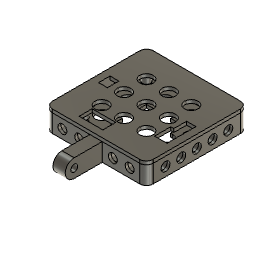
USB Camera Case v10 (Autodesk Fusion 360 design; units mm, degrees)
Autodesk Fusion 360 part; units mm, degrees
note: some values were not read from the file. Chosen so that the rebuilt part matches the saved one: which bodies a step acts on; which face or edge a step refers to. Set by a fixed rule: which sketch regions a step uses.
sketch "Camer Cutout" plane through (0, 0, 0) normal (0, 0, 1) x (1, 0, 0)
  line L0 (8.25, -8.25) -> (-8.25, -8.25)
  line L1 (-8.25, -8.25) -> (-8.25, 8.25)
  line L2 (-8.25, 8.25) -> (8.25, 8.25)
  line L3 (8.25, 8.25) -> (8.25, -8.25)
  line L4 (8.25, -8.25) -> (-8.25, 8.25) construction
  line L5 (-8.25, -8.25) -> (8.25, 8.25) construction
  arc A0 (8.25, -2.5) -> (8.25, 2.5) centre (8.25, 0) ccw
  arc A1 (-8.25, 2.5) -> (-8.25, -2.5) centre (-8.25, 0) ccw
  dimension "d1" = 16.5
  dimension "d2" = 16.5
  dimension "d3" = 2.5
  dimension "d4" = 2.5
  constraint horizontal L0
  constraint perpendicular L0 L1
  constraint parallel L0 L2
  constraint parallel L1 L3
  constraint coincident L4 origin
  constraint coincident L5 origin
  constraint midpoint L3 A0.centre
  constraint midpoint L1 A1.centre
  measures "d1" distance of L1.end L2.end
  measures "d2" distance of L0.end L1.end
  measures "d3" radius of A0
  measures "d4" radius of A1
sketch "Outer Standoff Lines" plane through (0, 0, 0) normal (0, 0, 1) x (1, 0, 0)
  line L0 (0, 0) -> (17, 0)
  line L1 (0, 0) -> (-17, 0)
  line L2 (-17, 0) -> (-17, 17)
  line L3 (-17, 0) -> (-17, -17)
  line L4 (17, 0) -> (17, -17)
  line L5 (17, 0) -> (17, 17)
  dimension "d5" = 17
  dimension "d6" = 17
  dimension "d7" = 17
  dimension "d8" = 17
  dimension "d9" = 17
  constraint coincident L0.start L1.start
  constraint horizontal L0
  constraint parallel L0 L1
  constraint perpendicular L1 L2
  constraint perpendicular L1 L3
  constraint perpendicular L0 L4
  constraint perpendicular L0 L5
  measures "d5" distance of L0.start L0.end
  measures "d6" distance of L1.end L2.end
  measures "d7" distance of L1.end L3.end
  measures "d8" distance of L0.end L4.end
  measures "d9" distance of L0.end L5.end
sketch "Inner Standoff Lines" plane through (0, 0, 0) normal (0, 0, 1) x (1, 0, 0)
  line L0 (0, 0) -> (14, 0)
  line L1 (14, 0) -> (14, -14)
  line L2 (14, 0) -> (14, 14)
  line L3 (0, 0) -> (-14, 0)
  line L4 (-14, 0) -> (-14, 14)
  line L5 (-14, 0) -> (-14, -14)
  dimension "d10" = 14
  dimension "d11" = 14
  dimension "d12" = 14
  dimension "d13" = 14
  dimension "d14" = 14
  dimension "d15" = 14
  constraint coincident L0.start L3.start
  constraint horizontal L0
  constraint perpendicular L0 L1
  constraint perpendicular L0 L2
  constraint perpendicular L2 L3
  constraint perpendicular L3 L4
  constraint perpendicular L3 L5
  measures "d10" distance of L0.start L0.end
  measures "d11" distance of L0.end L1.end
  measures "d12" distance of L0.end L2.end
  measures "d13" distance of L0.start L3.end
  measures "d14" distance of L3.end L4.end
  measures "d15" distance of L3.end L5.end
sketch "Outer Standoffs" plane through (0, 0, 0) normal (0, 0, 1) x (1, 0, 0)
  circle A0 centre (-17, 17) radius 1.1
  circle A1 centre (-17, -17) radius 1.1
  circle A2 centre (17, -17) radius 1.1
  circle A3 centre (17, 17) radius 1.1
  dimension "d16" = 2.2
  dimension "d17" = 2.2
  dimension "d18" = 2.2
  dimension "d19" = 2.2
  measures "d16" diameter of A0
  measures "d17" diameter of A1
  measures "d18" diameter of A2
  measures "d19" diameter of A3
sketch "Inner Standoffs" plane through (0, 0, 0) normal (0, 0, 1) x (1, 0, 0)
  circle A0 centre (-14, 14) radius 1.1
  circle A1 centre (-14, -14) radius 1.1
  circle A2 centre (14, -14) radius 1.1
  circle A3 centre (14, 14) radius 1.1
  dimension "d20" = 2.2
  dimension "d21" = 2.2
  dimension "d22" = 2.2
  dimension "d23" = 2.2
  measures "d20" diameter of A0
  measures "d21" diameter of A1
  measures "d22" diameter of A2
  measures "d23" diameter of A3
sketch "Inner Standoff Bases" plane through (0, 0, 0) normal (0, 0, 1) x (1, 0, 0)
  circle A0 centre (-14, 14) radius 1.75
  circle A1 centre (-14, -14) radius 1.75
  circle A2 centre (14, -14) radius 1.75
  circle A3 centre (14, 14) radius 1.75
  dimension "d24" = 3.5
  dimension "d25" = 3.5
  dimension "d26" = 3.5
  dimension "d27" = 3.5
  measures "d24" diameter of A0
  measures "d25" diameter of A1
  measures "d26" diameter of A2
  measures "d27" diameter of A3
sketch "Outer Standoff Bases" plane through (0, 0, 0) normal (0, 0, 1) x (1, 0, 0)
  circle A0 centre (-17, 17) radius 1.75
  circle A1 centre (-17, -17) radius 1.75
  circle A2 centre (17, -17) radius 1.75
  circle A3 centre (17, 17) radius 1.75
  dimension "d28" = 3.5
  dimension "d29" = 3.5
  dimension "d30" = 3.5
  dimension "d31" = 3.5
  measures "d28" diameter of A0
  measures "d29" diameter of A1
  measures "d30" diameter of A2
  measures "d31" diameter of A3
sketch "Board Cutout" plane through (0, 0, 0) normal (0, 0, 1) x (1, 0, 0)
  line L0 (19.15, 19.15) -> (-19.15, 19.15)
  line L1 (-19.15, 19.15) -> (-19.15, -19.15)
  line L2 (-19.15, -19.15) -> (19.15, -19.15)
  line L3 (19.15, -19.15) -> (19.15, 19.15)
  line L4 (19.15, 19.15) -> (-19.15, -19.15) construction
  line L5 (-19.15, 19.15) -> (19.15, -19.15) construction
  dimension "d32" = 38.3
  dimension "d33" = 38.3
  constraint horizontal L0
  constraint perpendicular L0 L1
  constraint parallel L0 L2
  constraint parallel L1 L3
  constraint coincident L4 origin
  constraint coincident L5 origin
  measures "d32" distance of L1.end L2.end
  measures "d33" distance of L0.end L1.end
sketch "Case Outer Footprint" plane through (0, 0, 0) normal (0, 0, 1) x (1, 0, 0)
  line L0 (19.5, -22.5) -> (-19.5, -22.5)
  line L1 (-22.5, -19.5) -> (-22.5, 19.5)
  line L2 (-19.5, 22.5) -> (19.5, 22.5)
  line L3 (22.5, 19.5) -> (22.5, -19.5)
  line L4 (22.5, -22.5) -> (-22.5, 22.5) construction
  line L5 (-22.5, -22.5) -> (22.5, 22.5) construction
  arc A0 (-19.5, 22.5) -> (-22.5, 19.5) centre (-19.5, 19.5) ccw
  arc A1 (-22.5, -19.5) -> (-19.5, -22.5) centre (-19.5, -19.5) ccw
  arc A2 (19.5, -22.5) -> (22.5, -19.5) centre (19.5, -19.5) ccw
  arc A3 (22.5, 19.5) -> (19.5, 22.5) centre (19.5, 19.5) ccw
  dimension "d34" = 45
  dimension "d35" = 45
  dimension "d36" = 3
  constraint horizontal L0
  constraint perpendicular L0 L1
  constraint parallel L0 L2
  constraint parallel L1 L3
  constraint coincident L4 origin
  constraint coincident L5 origin
  constraint coincident L4.end L2
  constraint coincident L4.end L1
  constraint tangent L2 A0
  constraint tangent L1 A0
  constraint coincident L5.start L1
  constraint coincident L5.start L0
  constraint tangent L1 A1
  constraint tangent L0 A1
  constraint equal A0 A1
  constraint coincident L4.start L0
  constraint coincident L4.start L3
  constraint tangent L0 A2
  constraint tangent L3 A2
  constraint equal A0 A2
  constraint coincident L5.end L3
  constraint coincident L5.end L2
  constraint tangent L3 A3
  constraint tangent L2 A3
  constraint equal A0 A3
  measures "d34" distance of L4.end L5.end
  measures "d35" distance of L5.start L4.end
  measures "d36" radius of A0
sketch "Port 2 Cutout" plane through (0, 0, 0) normal (0, 0, 1) x (1, 0, 0)
  line L0 (-14, -14) -> (-10.5, -14)
  line L1 (-10.5, -14) -> (-10.5, -19.15)
  line L2 (-10.5, -19.15) -> (-10.5, -14.25)
  line L3 (-10.5, -14.25) -> (-0.35, -14.25)
  line L4 (-0.35, -14.25) -> (-0.35, -19.15)
  line L5 (-0.35, -19.15) -> (-10.5, -19.15)
  dimension "d37" = 3.5
  dimension "d38" = 5.15
  dimension "d39" = 4.9
  dimension "d40" = 10.15
  dimension "d41" = 4.9
  constraint horizontal L0
  constraint vertical L1
  constraint perpendicular L0 L2
  constraint perpendicular L2 L3
  constraint perpendicular L3 L4
  measures "d37" distance of L0.start L0.end
  measures "d38" distance of L0.end L1.end
  measures "d39" distance of L1.end L2.end
  measures "d40" distance of L2.end L3.end
  measures "d41" distance of L3.end L4.end
sketch "Port 1 Cutout" plane through (0, 0, 0) normal (0, 0, 1) x (1, 0, 0)
  line L0 (-14, -14) -> (-14, -1.8)
  line L1 (-14, -1.8) -> (-19.15, -1.8)
  line L2 (-19.15, -1.8) -> (-19.15, 2.9)
  line L3 (-19.15, 2.9) -> (-15.65, 2.9)
  line L4 (-15.65, 2.9) -> (-15.65, -1.8)
  dimension "d42" = 12.2
  dimension "d43" = 5.15
  dimension "d44" = 4.7
  dimension "d45" = 3.5
  constraint vertical L0
  constraint perpendicular L0 L1
  constraint perpendicular L1 L2
  constraint perpendicular L2 L3
  constraint coincident L1 L4.end
  constraint perpendicular L1 L4
  measures "d42" distance of L0.start L0.end
  measures "d43" distance of L0.end L1.end
  measures "d44" distance of L1.end L2.end
  measures "d45" distance of L2.end L3.end
sketch "Ports 3/4 Cutout" plane through (0, 0, 0) normal (0, 0, 1) x (1, 0, 0)
  line L0 (14, -14) -> (14, -10)
  line L1 (14, -10) -> (19.15, -10)
  line L2 (14, -10) -> (14, -3)
  line L3 (19.15, -10) -> (19.15, 2.5)
  line L4 (14, -3) -> (15.4, -3)
  line L5 (15.4, -3) -> (15.4, 2.5)
  line L6 (15.4, 2.5) -> (19.15, 2.5)
  dimension "d46" = 4
  dimension "d47" = 5.15
  dimension "d48" = 7
  dimension "d49" = 12.5
  dimension "d50" = 1.4
  constraint vertical L0
  constraint perpendicular L0 L1
  constraint perpendicular L1 L2
  constraint perpendicular L1 L3
  constraint perpendicular L2 L4
  constraint perpendicular L4 L5
  constraint perpendicular L3 L6
  measures "d46" distance of L0.start L0.end
  measures "d47" distance of L0.end L1.end
  measures "d48" distance of L0.end L2.end
  measures "d49" distance of L1.end L3.end
  measures "d50" distance of L2.end L4.end
sketch "Back Insert Footprint" plane through (0, 0, 0) normal (0, 0, 1) x (1, 0, 0)
  line L0 (18.75, 21.25) -> (-18.75, 21.25)
  line L1 (-21.25, 18.75) -> (-21.25, -18.75)
  line L2 (-18.75, -21.25) -> (18.75, -21.25)
  line L3 (21.25, -18.75) -> (21.25, 18.75)
  line L4 (21.25, 21.25) -> (-21.25, -21.25) construction
  line L5 (-21.25, 21.25) -> (21.25, -21.25) construction
  arc A0 (-18.75, 21.25) -> (-21.25, 18.75) centre (-18.75, 18.75) ccw
  arc A1 (-21.25, -18.75) -> (-18.75, -21.25) centre (-18.75, -18.75) ccw
  arc A2 (18.75, -21.25) -> (21.25, -18.75) centre (18.75, -18.75) ccw
  arc A3 (21.25, 18.75) -> (18.75, 21.25) centre (18.75, 18.75) ccw
  dimension "d51" = 42.5
  dimension "d52" = 42.5
  dimension "d53" = 2.5
  constraint horizontal L0
  constraint perpendicular L0 L1
  constraint parallel L0 L2
  constraint parallel L1 L3
  constraint coincident L4 origin
  constraint coincident L5 origin
  constraint coincident L5.start L0
  constraint coincident L5.start L1
  constraint tangent L0 A0
  constraint tangent L1 A0
  constraint coincident L4.end L1
  constraint coincident L4.end L2
  constraint tangent L1 A1
  constraint tangent L2 A1
  constraint equal A0 A1
  constraint coincident L5.end L2
  constraint coincident L5.end L3
  constraint tangent L2 A2
  constraint tangent L3 A2
  constraint equal A0 A2
  constraint coincident L4.start L3
  constraint coincident L4.start L0
  constraint tangent L3 A3
  constraint tangent L0 A3
  constraint equal A0 A3
  measures "d51" distance of L4.end L5.end
  measures "d52" distance of L5.start L4.end
  measures "d53" radius of A0
extrude "Extrude1" add sketch "Case Outer Footprint" along normal blind 8 makes body 1
extrude "Extrude2" cut sketch "Back Insert Footprint" along normal blind 20 from surface at 1.5 bodies 1
extrude "Extrude3" cut sketch "Camer Cutout" along normal blind 5 bodies 1
extrude "Extrude4" add sketch "Outer Standoff Bases" sketch "Inner Standoff Bases" along normal blind 3 of sketch 2 bodies 1
extrude "Extrude5" add sketch "Inner Standoffs" sketch "Outer Standoffs" along normal blind 5.5 of sketch 2 bodies 1
extrude "Extrude6" add sketch "Outer Standoff Bases" sketch "Inner Standoff Bases" along normal blind 3.3 from surface at 4.7 separate body of sketch 2 makes body 2 at (-12.2587, 13.8258, 5.8) makes body 3 at (15.7413, 13.8258, 5.8) makes body 4 at (-15.2587, 16.8258, 5.8) makes body 5 at (18.7413, 16.8258, 5.8) makes body 6 at (-15.2587, -17.1742, 5.8) makes body 7 at (18.7413, -17.1742, 5.8) makes body 8 at (-12.2587, -14.1742, 5.8) makes body 9 at (15.7413, -14.1742, 5.8)
extrude "Extrude7" add sketch "Case Outer Footprint" along normal blind 1.5 from surface at 8 bodies 2 3 4 5 6 7 8 9
extrude "Extrude8" cut sketch "Inner Standoffs" sketch "Outer Standoffs" along normal blind 5.5 of sketch 2 bodies 2
extrude "Extrude9" cut sketch "Ports 3/4 Cutout" sketch "Port 1 Cutout" sketch "Port 2 Cutout" along normal blind 10 of sketch 2 of sketch 3 bodies 2
extrude "Extrude10" add sketch "Back Insert Footprint" sketch "Board Cutout" along normal blind 8 separate body of sketch 2 makes body 10
extrude "Extrude11" cut sketch "Board Cutout" along normal blind 8 bodies 10
extrude "Extrude12" cut sketch "Back Insert Footprint" along normal blind 1.5 bodies 10
combine "Combine1" operation add target body 2 tool bodies 10
sketch "Mount Arm" plane through (0, 0, 0) normal (1, 0, 0) x (0, 1, 0)
  line L0 (-22.5, 0) -> (-22.5, 8)
  line L1 (-22.5, 8) -> (-35, 8)
  line L2 (-22.5, 0) -> (-35, 0)
  arc A0 (-35, 8) -> (-35, 0) centre (-35, 4) ccw
  circle A1 centre (-35, 4) radius 1.525
  dimension "d81" = 3.05
  constraint vertical L0
  constraint perpendicular L0 L1
  constraint perpendicular L0 L2
  constraint concentric A0 A1
  measures "d81" diameter of A1
extrude "Extrude13" add sketch "Mount Arm" along normal mid plane 5.5 bodies 1
sketch "Frame Cutout" plane through (0, 0, 0) normal (0, 0, 1) x (1, 0, 0)
  line L0 (0, 0) -> (-22, 22)
  circle A0 centre (-10, 10) radius 3
  circle A1 centre (0, 10) radius 3
  circle A2 centre (10, 10) radius 3
  circle A3 centre (-10, 0) radius 3
  circle A4 centre (0, 0) radius 3
  circle A5 centre (10, 0) radius 3
  circle A6 centre (-10, -10) radius 3
  circle A7 centre (0, -10) radius 3
  circle A8 centre (10, -10) radius 3
  dimension "d86" = 20
  dimension "d87" = -20
  constraint coincident L0.start A4.centre
  constraint coincident L0 A0.centre
extrude "Extrude14" cut sketch "Frame Cutout" along normal blind 20 bodies 2
sketch "Side Cutout" plane through (22.5, 0, 0) normal (1, 0, 0) x (0, 1, 0)
  line L0 (-19.5, 0) -> (19.5, 0)
  line L1 (19.5, 0) -> (19.5, 8)
  line L2 (19.5, 8) -> (-19.5, 8)
  line L3 (-19.5, 8) -> (-19.5, 0)
  line L4 (0, 8) -> (0, 0)
  line L5 (0, 0) -> (0, 4)
  circle A0 centre (0, 4) radius 2
  circle A1 centre (-14, 4) radius 2
  circle A2 centre (-7, 4) radius 2
  circle A3 centre (7, 4) radius 2
  circle A4 centre (14, 4) radius 2
  dimension "d92" = 4
  dimension "d95" = 14
  dimension "d96" = 0
  constraint midpoint L2 L4.start
  constraint coincident L4.end L5.start
  constraint midpoint L4 L5.end
  measures "d92" diameter of A0
extrude "Extrude16" cut sketch "Side Cutout" against normal blind 3.5 contours L4 L5 A0 | L4 L5 A0 | A1 | A2 | A3 | A4 bodies 1 2
extrude "Extrude17" cut sketch "Side Cutout" against normal blind 28 from surface at -41 contours L4 L5 A0 | L4 L5 A0 | A1 | A2 | A3 | A4 bodies 1 2
sketch "Top Cutout" plane through (0, 22.5, 0) normal (0, 1, 0) x (-1, 0, 0)
  line L0 (-19.5, 0) -> (19.5, 0)
  line L1 (19.5, 0) -> (19.5, 8)
  line L2 (19.5, 8) -> (-19.5, 8)
  line L3 (-19.5, 8) -> (-19.5, 0)
  line L4 (0, 0) -> (0, 8)
  line L5 (0, 0) -> (0, 4)
  circle A0 centre (0, 4) radius 2
  circle A1 centre (-15, 4) radius 2
  circle A2 centre (-7.5, 4) radius 2
  circle A3 centre (7.5, 4) radius 2
  circle A4 centre (15, 4) radius 2
  dimension "d102" = 4
  dimension "d105" = 15
  dimension "d106" = 0
  constraint coincident L4.start L5.start
  constraint midpoint L2 L4.end
  constraint midpoint L4 L5.end
  measures "d102" diameter of A0
extrude "Extrude18" cut sketch "Top Cutout" against normal blind 3.5 contours L4 L5 A0 | L4 L5 A0 | A1 | A2 | A3 | A4 bodies 1 2
extrude "Extrude19" cut sketch "Top Cutout" along normal blind 10 from surface at -51.5 contours A1 | A2 | A3 | A4 bodies 1 2
sketch "Sketch18" plane through (0, 0, 0) normal (0, 0, 1) x (1, 0, 0)
  circle A0 centre (0, 0) radius 17
  line L0 (0, 0) -> (0, -17)
  line L1 (0, 0) -> (-8.6104, -20.7873)
  circle A1 centre (-5.8168, -14.043) radius 3
  circle A2 centre (5.8168, -14.043) radius 3
  circle A3 centre (14.043, -5.8168) radius 3
  circle A4 centre (14.043, 5.8168) radius 3
  circle A5 centre (5.8168, 14.043) radius 3
  circle A6 centre (-5.8168, 14.043) radius 3
  circle A7 centre (-14.043, 5.8168) radius 3
  circle A8 centre (-14.043, -5.8168) radius 3
  dimension "d112" = 157.5
  dimension "d113" = 22.5
  dimension "d114" = 6
  dimension "d116" = 360
  constraint coincident A0.centre L0.start
  constraint coincident A0 L0.end
  constraint vertical L0
  constraint coincident L1 A1.centre
  measures "d112" angle of L0 L1
  measures "d113" distance of A0.centre L1.end
  measures "d114" diameter of A1
extrude "Extrude20" cut sketch "Sketch18" along normal blind 5 contours A0 A4 | A0 A4 | A0 A3 | A0 A3 | A0 A5 | A0 A5 | A0 A2 | A0 A2 | A0 A6 | A0 A6 | A0 L1 A1 | A0 L1 A1 | A0 A7 | A0 A7 | A0 L1 A1 | A0 L1 A1 | A0 A8 | A0 A8 bodies 1
chamfer "Chamfer1" distance 0.4 angle 45 8 edges at (21.25, 0, 1.5) (20.5178, 20.5178, 1.5) (0, 21.25, 1.5) (-20.5178, 20.5178, 1.5) (-21.25, 0, 1.5) (-20.5178, -20.5178, 1.5) (0, -21.25, 1.5) (20.5178, -20.5178, 1.5) on bodies 2
fillet "Fillet1" radius 0.2 8 edges at (-21.25, 0, 1.9) (-20.5178, 20.5178, 1.9) (0, 21.25, 1.9) (20.5178, 20.5178, 1.9) (21.25, 0, 1.9) (20.5178, -20.5178, 1.9) (0, -21.25, 1.9) (-20.5178, -20.5178, 1.9) on bodies 2
extrude "Extrude21" cut 1 faces at (-7.1167, -14.25, 8.5) along direction (0, 1, 0) blind 0.5 on bodies 2 bodies 2
extrude "Extrude22" cut 8 faces at (15.5227, 13.8584, 4.7) (18.5268, 16.9131, 4.7) (18.5227, -17.1416, 4.7) (15.5227, -14.1416, 4.7) (-15.4773, -17.1416, 4.7) (-12.4773, -14.1416, 4.7) (-12.4773, 13.8584, 4.7) (-15.4732, 16.9131, 4.7) along direction (0, 0, 1) blind 0.05 on bodies 2 bodies 2
sketch "Sketch19" plane through (0, 0, 0) normal (0, 0, 1) x (1, 0, 0)
  line L0 (8.25, 2.5) -> (8.25, -2.5)
  line L1 (8.25, -2.5) -> (9.25, -2.5)
  line L2 (9.25, -2.5) -> (9.25, 2.5)
  line L3 (9.25, 2.5) -> (8.25, 2.5)
  line L4 (-8.25, -2.5) -> (-8.25, 2.5)
  line L5 (-8.25, 2.5) -> (-9.25, 2.5)
  line L6 (-9.25, 2.5) -> (-9.25, -2.5)
  line L7 (-9.25, -2.5) -> (-8.25, -2.5)
  arc A0 (-9.25, 2.5) -> (-9.25, -2.5) centre (-9.25, 0) ccw
  arc A1 (9.25, -2.5) -> (9.25, 2.5) centre (9.25, 0) ccw
  line L8 (0, -9.25) -> (2.5, -9.25)
  line L9 (0, -9.25) -> (-2.5, -9.25)
  arc A2 (-2.5, -9.25) -> (2.5, -9.25) centre (0, -9.25) ccw
  line L10 (2.5, -9.25) -> (2.5, -8.25)
  line L11 (-2.5, -9.25) -> (-2.5, -8.25)
  line L12 (-2.5, -8.25) -> (2.5, -8.25)
  line L13 (0, 9.25) -> (2.5, 9.25)
  line L14 (0, 9.25) -> (-2.5, 9.25)
  line L15 (-2.5, 9.25) -> (-2.5, 8.25)
  line L16 (2.5, 9.25) -> (2.5, 8.25)
  line L17 (2.5, 8.25) -> (-2.5, 8.25)
  arc A3 (2.5, 9.25) -> (-2.5, 9.25) centre (0, 9.25) ccw
  dimension "d125" = 1
  dimension "d126" = 1
  dimension "d160" = 2.5
  dimension "d161" = 2.5
  dimension "d162" = 1
  dimension "d165" = 2.5
  dimension "d166" = 2.5
  dimension "d167" = 1
  dimension "d168" = 1
  constraint vertical L0
  constraint perpendicular L0 L1
  constraint perpendicular L1 L2
  constraint perpendicular L0 L3
  constraint perpendicular L1 L4
  constraint perpendicular L4 L5
  constraint perpendicular L5 L6
  constraint perpendicular L4 L7
  constraint tangent L5 A0
  constraint tangent L3 A1
  constraint coincident L8.start L9.start
  constraint perpendicular L8 L10
  constraint tangent A2 L11
  constraint perpendicular L10 L12
  constraint perpendicular L14 L15
  constraint perpendicular L13 L16
  constraint coincident L13.start L14.start
  measures "d125" distance of L0.end L1.end
  measures "d126" distance of L4.end L5.end
  measures "d160" distance of L8.start L8.end
  measures "d161" distance of L8.start L9.end
  measures "d162" distance of L8.end L10.end
  measures "d165" distance of L13.start L13.end
  measures "d166" distance of L13.start L14.end
  measures "d167" distance of L14.end L15.end
  measures "d168" distance of L13.end L16.end
extrude "Extrude23" cut sketch "Sketch19" along normal blind 1.5 bodies 1
chamfer "Chamfer2" distance 0.1 angle 45 8 edges at (-15.0256, 13.6022, 5.5) (-18.0256, 16.6022, 5.5) (-18.0256, -17.3978, 5.5) (-15.0256, -14.3978, 5.5) (15.9744, -17.3978, 5.5) (12.9744, -14.3978, 5.5) (12.9744, 13.6022, 5.5) (15.9744, 16.6022, 5.5) on bodies 1
extrude "Extrude24" cut 1 faces at (-10.5, -17.35, 8.5) along direction (-1, 0, 0) blind 0.2 on bodies 2 bodies 2
extrude "Extrude25" cut 1 faces at (-0.35, -15.55, 9) along direction (1, 0, 0) blind 0.2 on bodies 2 bodies 2
extrude "Extrude26" cut 1 faces at (-3.6667, -13.75, 8.5) along direction (0, 1, 0) blind 0.2 on bodies 2 bodies 2
extrude "Extrude27" cut 1 faces at (-17.9833, 2.9, 8.5) along direction (0, 1, 0) blind 0.2 on bodies 2 bodies 2
extrude "Extrude28" cut 1 faces at (-15.65, 1.4667, 8.5) along direction (1, 0, 0) blind 0.2 on bodies 2 bodies 2
extrude "Extrude29" cut 1 faces at (-16.6833, -1.8, 8.5) along direction (0, -1, 0) blind 0.2 on bodies 2 bodies 2
extrude "Extrude30" cut 1 faces at (15.7167, -10, 8.5) along direction (0, -1, 0) blind 0.2 on bodies 2 bodies 2
extrude "Extrude31" cut 1 faces at (16.65, 2.5, 8.5) along direction (0, 1, 0) blind 0.2 on bodies 2 bodies 2
extrude "Extrude32" cut 1 faces at (15.4, -1.1, 8.5) along direction (-1, 0, 0) blind 0.2 on bodies 2 bodies 2
extrude "Extrude33" cut 1 faces at (14, -7.8, 8.5) along direction (-1, 0, 0) blind 0.2 on bodies 2 bodies 2
extrude "Extrude34" cut 2 faces at (19.15, -18.0926, 4.5994) (19.15, -1.6, 8.5) along direction (1, 0, 0) blind 0.2 on bodies 2 bodies 2
extrude "Extrude35" cut 2 faces at (-19.15, 18.0926, 4.5994) (-19.15, -0.3, 8.5) along direction (-1, 0, 0) blind 0.2 on bodies 2 bodies 2
extrude "Extrude36" cut 1 faces at (18.5592, 19.15, 4.5994) along direction (0, 1, 0) blind 0.2 on bodies 2 bodies 2
extrude "Extrude37" cut 2 faces at (-0.05, -19.15, 5.1346) (-3.6667, -19.15, 8.5) along direction (0, -1, 0) blind 0.2 on bodies 2 bodies 2
extrude "Extrude38" cut sketch "Top Cutout" against normal blind 65 contours L4 L5 A0 | L4 L5 A0 bodies 2
equation "d107 = 0 mm - 3.500 mm"
equation "d112 = 180 deg - 22.5 deg"
named bodies: "USB Camera Case (Front)", "USB Camera Case (Back)"
